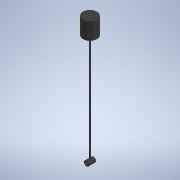
# Autodesk Inventor part: pendulumSimple
Saved by Autodesk Inventor 2020 (Build 240168000, 168)
## iProperties
Created: 2020-06-14
Part Number: pendulumSimple
Material: Steel
Document SubType Name: Modeling
Designer: Freeman
Mass: 1.01129e+06 g
Surface Area: 21938.6 cm^2
Volume: 128827 cm^3
Density: 7.85 g/cm^3
Appearance: Plate
Author: Freeman
Autodesk Inventor part; units mm, degrees
ref_plane "YZ Plane" through (0, 0, 0) normal (1, 0, 0) x (0, 1, 0)
ref_plane "XZ Plane" through (0, 0, 0) normal (0, 1, 0) x (-1, 0, 0)
ref_plane "XY Plane" through (0, 0, 0) normal (0, 0, 1) x (1, 0, 0)
sketch "Sketch4" plane through (0, 0, 0) normal (0, 0, 1) x (1, 0, 0)
  circle A0 centre (0, 0) radius 60
  circle A1 centre (0, 0) radius 90
  dimension "d14" = 120
  dimension "d15" = 180
  constraints: 2 centre point, 2 coincident
  measures "d14" diameter of A0
  measures "d15" diameter of A1
extrude "Extrusion2" add sketch "Sketch4" along normal mid plane 250
sketch "Sketch6" plane through (0, 0, 0) normal (0, 1, 0) x (-1, 0, 0)
  circle A0 centre (0, 0) radius 25
  dimension "d18" = 50
  constraints: 1 centre point, 1 coincident
  measures "d18" diameter of A0
extrude "Extrusion3" add sketch "Sketch6" along normal blind 4500
sketch "Sketch7" plane through (0, 0, 125) normal (0, 0, 1) x (1, 0, 0)
  point P0 (0, 0)
  point P1 (0, 0)
  constraints: 1 coincident
hole "Hole1" at (0, 0, 125) direction (0, 0, -1) diameter 120 end through all
sketch "Sketch8" plane through (0, 4500, 0) normal (0, 1, 0) x (1, 0, 0)
  circle A0 centre (0, 0) radius 250
  dimension "d28" = 500
  constraints: 1 centre point, 1 coincident
  measures "d28" diameter of A0
extrude "Extrusion4" add sketch "Sketch8" against normal blind 600
body "Solid2"
